Autodesk Inventor part; units mm, degrees
(part 2 of 2)
  line L317 (12.3467, 21.5941) -> (15.1117, 21.5941)
  line L318 (-7.2627, 18.1267) -> (-7.2627, 11.634)
  line L319 (-3.9937, 18.1267) -> (-7.2627, 18.1267)
  line L320 (-3.9937, 11.634) -> (-3.9937, 18.1267)
  line L321 (-7.2627, 11.634) -> (-3.9937, 11.634)
  line L322 (2.8777, 19.9119) -> (2.8777, 17.0508)
  line L323 (5.6982, 19.9119) -> (2.8777, 19.9119)
  line L324 (5.6982, 17.0508) -> (5.6982, 19.9119)
  line L325 (2.8777, 17.0508) -> (5.6982, 17.0508)
  line L326 (6.6317, 14.6767) -> (6.6317, 13.9462)
  line L327 (8.2279, 14.6767) -> (6.6317, 14.6767)
  line L328 (8.2279, 13.9462) -> (8.2279, 14.6767)
  line L329 (6.6317, 13.9462) -> (8.2279, 13.9462)
  line L330 (-11.4396, 26.1143) -> (-11.4396, 21.5941)
  line L331 (-8.2765, 26.1143) -> (-11.4396, 26.1143)
  line L332 (-8.2765, 21.5941) -> (-8.2765, 26.1143)
  line L333 (-11.4396, 21.5941) -> (-8.2765, 21.5941)
  line L334 (23.7979, 4.6422) -> (23.7979, 3.9161)
  line L335 (25.3456, 4.6422) -> (23.7979, 4.6422)
  line L336 (25.3456, 3.9161) -> (25.3456, 4.6422)
  line L337 (23.7979, 3.9161) -> (25.3456, 3.9161)
  line L338 (25.9674, 12.5506) -> (25.9674, 11.0937)
  line L339 (26.969, 12.5506) -> (25.9674, 12.5506)
  line L340 (26.969, 11.0937) -> (26.969, 12.5506)
  line L341 (25.9674, 11.0937) -> (26.969, 11.0937)
  line L342 (20.5866, 13.4064) -> (20.5866, 10.1468)
  line L343 (22.4384, 13.4064) -> (20.5866, 13.4064)
  line L344 (22.4384, 10.1468) -> (22.4384, 13.4064)
  line L345 (20.5866, 10.1468) -> (22.4384, 10.1468)
  line L346 (13.1069, 19.0982) -> (13.1069, 18.337)
  line L347 (14.6707, 19.0982) -> (13.1069, 19.0982)
  line L348 (14.6707, 18.337) -> (14.6707, 19.0982)
  line L349 (13.1069, 18.337) -> (14.6707, 18.337)
  line L350 (-2.8376, 26.8483) -> (-2.8376, 26.1143)
  line L351 (-1.3678, 26.8483) -> (-2.8376, 26.8483)
  line L352 (-1.3678, 26.1143) -> (-1.3678, 26.8483)
  line L353 (-2.8376, 26.1143) -> (-1.3678, 26.1143)
  line L354 (3.5053, 26.9808) -> (3.5053, 26.1143)
  line L355 (5.0811, 26.9808) -> (3.5053, 26.9808)
  line L356 (5.0811, 26.1143) -> (5.0811, 26.9808)
  line L357 (3.5053, 26.1143) -> (5.0811, 26.1143)
  line L358 (9.7366, 26.9808) -> (9.7366, 26.1143)
  line L359 (11.3, 26.9808) -> (9.7366, 26.9808)
  line L360 (11.3, 26.1143) -> (11.3, 26.9808)
  line L361 (9.7366, 26.1143) -> (11.3, 26.1143)
  line L362 (12.7922, 32.175) -> (12.7922, 30.9022)
  line L363 (14.5702, 32.175) -> (12.7922, 32.175)
  line L364 (14.5702, 30.9022) -> (14.5702, 32.175)
  line L365 (12.7922, 30.9022) -> (14.5702, 30.9022)
  line L366 (13.3079, 38.2648) -> (13.3079, 35.0088)
  line L367 (14.1615, 38.2648) -> (13.3079, 38.2648)
  line L368 (14.1615, 35.0088) -> (14.1615, 38.2648)
  line L369 (13.3079, 35.0088) -> (14.1615, 35.0088)
  line L370 (12.9292, 42.1098) -> (12.9292, 41.3551)
  line L371 (14.3655, 42.1098) -> (12.9292, 42.1098)
  line L372 (14.3655, 41.3551) -> (14.3655, 42.1098)
  line L373 (12.9292, 41.3551) -> (14.3655, 41.3551)
  line L374 (-2.9701, 39.8497) -> (-2.9701, 39.0772)
  line L375 (-1.3678, 39.8497) -> (-2.9701, 39.8497)
  line L376 (-1.3678, 39.0772) -> (-1.3678, 39.8497)
  line L377 (-2.9701, 39.0772) -> (-1.3678, 39.0772)
  line L378 (-2.6721, 35.9046) -> (-2.6721, 32.7312)
  line L379 (-1.7091, 35.9046) -> (-2.6721, 35.9046)
  line L380 (-1.7091, 32.7312) -> (-1.7091, 35.9046)
  line L381 (-2.6721, 32.7312) -> (-1.7091, 32.7312)
  line L382 (61.5532, 35.0088) -> (61.5532, 33.5887)
  line L383 (63.3578, 35.0088) -> (61.5532, 35.0088)
  line L384 (63.3578, 33.5887) -> (63.3578, 35.0088)
  line L385 (61.5532, 33.5887) -> (63.3578, 33.5887)
  line L386 (-2.3, 45.1616) -> (-2.3, 41.9097)
  line L387 (-0.4798, 45.1616) -> (-2.3, 45.1616)
  line L388 (-0.4798, 41.9097) -> (-0.4798, 45.1616)
  line L389 (-2.3, 41.9097) -> (-0.4798, 41.9097)
  arc A22 (0.3948, 25.0132) -> (0.3948, 21.2543) centre (0.717, 23.1338) ccw
  line L390 (8.2935, 25.0132) -> (0.3948, 25.0132)
  arc A23 (8.2935, 21.2543) -> (8.2935, 25.0132) centre (7.9713, 23.1338) ccw
  line L391 (0.3948, 21.2543) -> (8.2935, 21.2543)
  circle A24 centre (11.0964, 6.0607) radius 3.302
  line L392 (53.7966, 24.6667) -> (53.7966, 25.3313)
  line L393 (52.7806, 23.6507) -> (53.7966, 24.6667)
  line L394 (49.402, 23.6507) -> (52.7806, 23.6507)
  line L395 (48.386, 24.6667) -> (49.402, 23.6507)
  line L396 (48.386, 25.3313) -> (48.386, 24.6667)
  line L397 (49.402, 26.3473) -> (48.386, 25.3313)
  line L398 (52.7806, 26.3473) -> (49.402, 26.3473)
  line L399 (53.7966, 25.3313) -> (52.7806, 26.3473)
  line L400 (1.7827, 46.235) -> (1.1223, 46.235)
  line L401 (2.7987, 45.219) -> (1.7827, 46.235)
  line L402 (2.7987, 41.8408) -> (2.7987, 45.219)
  line L403 (1.7827, 40.8248) -> (2.7987, 41.8408)
  line L404 (1.1223, 40.8248) -> (1.7827, 40.8248)
  line L405 (0.1063, 41.8408) -> (1.1223, 40.8248)
  line L406 (0.1063, 45.219) -> (0.1063, 41.8408)
  line L407 (1.1223, 46.235) -> (0.1063, 45.219)
  line L408 (6.7103, 46.235) -> (5.6943, 45.219)
  line L409 (7.3707, 46.235) -> (6.7103, 46.235)
  line L410 (8.3867, 45.219) -> (7.3707, 46.235)
  line L411 (8.3867, 41.8408) -> (8.3867, 45.219)
  line L412 (7.3707, 40.8248) -> (8.3867, 41.8408)
  line L413 (6.7103, 40.8248) -> (7.3707, 40.8248)
  line L414 (5.6943, 41.8408) -> (6.7103, 40.8248)
  line L415 (5.6943, 45.219) -> (5.6943, 41.8408)
  circle A25 centre (0, 48.3362) radius 1.5621
  circle A26 centre (0, 0) radius 1.5621
  circle A27 centre (82.6262, 0) radius 1.5621
  circle A28 centre (51.6255, 4.8785) radius 1.5621
  circle A29 centre (51.6255, 32.8947) radius 1.3153
  circle A30 centre (75.1332, 48.3362) radius 1.5621
  line L416 (3.9163, 46.235) -> (2.9003, 45.219)
  line L417 (4.5767, 46.235) -> (3.9163, 46.235)
  line L418 (5.5927, 45.219) -> (4.5767, 46.235)
  line L419 (5.5927, 41.8408) -> (5.5927, 45.219)
  line L420 (4.5767, 40.8248) -> (5.5927, 41.8408)
  line L421 (3.9163, 40.8248) -> (4.5767, 40.8248)
  line L422 (2.9003, 41.8408) -> (3.9163, 40.8248)
  line L423 (2.9003, 45.219) -> (2.9003, 41.8408)
  line L424 (53.7966, 21.8727) -> (53.7966, 22.5373)
  line L425 (52.7806, 20.8567) -> (53.7966, 21.8727)
  line L426 (49.402, 20.8567) -> (52.7806, 20.8567)
  line L427 (48.386, 21.8727) -> (49.402, 20.8567)
  line L428 (48.386, 22.5373) -> (48.386, 21.8727)
  line L429 (49.402, 23.5533) -> (48.386, 22.5373)
  line L430 (52.7806, 23.5533) -> (49.402, 23.5533)
  line L431 (53.7966, 22.5373) -> (52.7806, 23.5533)
  line L432 (53.7966, 27.4607) -> (53.7966, 28.1253)
  line L433 (52.7806, 26.4447) -> (53.7966, 27.4607)
  line L434 (49.402, 26.4447) -> (52.7806, 26.4447)
  line L435 (48.386, 27.4607) -> (49.402, 26.4447)
  line L436 (48.386, 28.1253) -> (48.386, 27.4607)
  line L437 (49.402, 29.1413) -> (48.386, 28.1253)
  line L438 (52.7806, 29.1413) -> (49.402, 29.1413)
  line L439 (53.7966, 28.1253) -> (52.7806, 29.1413)
  circle A31 centre (3.9075, 6.0607) radius 3.302
  line L440 (57.1918, 28.2371) -> (57.1918, 21.9581)
  line L441 (63.6527, 28.2371) -> (57.1918, 28.2371)
  line L442 (63.6527, 21.9581) -> (63.6527, 28.2371)
  line L443 (57.1918, 21.9581) -> (63.6527, 21.9581)
  line L444 (66.3035, 35.9046) -> (66.3035, 32.5006)
  line L445 (67.5508, 35.9046) -> (66.3035, 35.9046)
  line L446 (67.5508, 32.5006) -> (67.5508, 35.9046)
  line L447 (66.3035, 32.5006) -> (67.5508, 32.5006)
  line L448 (-2.9701, 32.0256) -> (-2.9701, 31.0896)
  line L449 (-1.3678, 32.0256) -> (-2.9701, 32.0256)
  line L450 (-1.3678, 31.0896) -> (-1.3678, 32.0256)
  line L451 (-2.9701, 31.0896) -> (-1.3678, 31.0896)
  line L452 (-2.9701, 37.5322) -> (-2.9701, 36.6368)
  line L453 (-1.3678, 37.5322) -> (-2.9701, 37.5322)
  line L454 (-1.3678, 36.6368) -> (-1.3678, 37.5322)
  line L455 (-2.9701, 36.6368) -> (-1.3678, 36.6368)
  line L456 (-6.9964, 42.9992) -> (-6.9964, 41.9097)
  line L457 (-5.0545, 42.9992) -> (-6.9964, 42.9992)
  line L458 (-5.0545, 41.9097) -> (-5.0545, 42.9992)
  line L459 (-6.9964, 41.9097) -> (-5.0545, 41.9097)
  line L460 (12.7922, 40.0541) -> (12.7922, 38.8221)
  line L461 (14.5702, 40.0541) -> (12.7922, 40.0541)
  line L462 (14.5702, 38.8221) -> (14.5702, 40.0541)
  line L463 (12.7922, 38.8221) -> (14.5702, 38.8221)
  line L464 (12.7922, 34.4881) -> (12.7922, 33.2287)
  line L465 (14.5702, 34.4881) -> (12.7922, 34.4881)
  line L466 (14.5702, 33.2287) -> (14.5702, 34.4881)
  line L467 (12.7922, 33.2287) -> (14.5702, 33.2287)
  line L468 (13.3079, 29.9286) -> (13.3079, 26.7098)
  line L469 (14.3655, 29.9286) -> (13.3079, 29.9286)
  line L470 (14.3655, 26.7098) -> (14.3655, 29.9286)
  line L471 (13.3079, 26.7098) -> (14.3655, 26.7098)
  line L472 (6.6317, 26.9808) -> (6.6317, 26.1143)
  line L473 (8.1119, 26.9808) -> (6.6317, 26.9808)
  line L474 (8.1119, 26.1143) -> (8.1119, 26.9808)
  line L475 (6.6317, 26.1143) -> (8.1119, 26.1143)
  line L476 (0.2905, 26.8483) -> (0.2905, 26.1143)
  line L477 (1.8236, 26.8483) -> (0.2905, 26.8483)
  line L478 (1.8236, 26.1143) -> (1.8236, 26.8483)
  line L479 (0.2905, 26.1143) -> (1.8236, 26.1143)
  line L480 (-2.9701, 28.4771) -> (-2.9701, 27.8018)
  line L481 (-1.3678, 28.4771) -> (-2.9701, 28.4771)
  line L482 (-1.3678, 27.8018) -> (-1.3678, 28.4771)
  line L483 (-2.9701, 27.8018) -> (-1.3678, 27.8018)
  line L484 (13.0148, 15.7926) -> (13.0148, 15.0444)
  line L485 (14.5702, 15.7926) -> (13.0148, 15.7926)
  line L486 (14.5702, 15.0444) -> (14.5702, 15.7926)
  line L487 (13.0148, 15.0444) -> (14.5702, 15.0444)
  line L488 (23.6729, 13.4064) -> (23.6729, 10.1468)
  line L489 (24.9476, 13.4064) -> (23.6729, 13.4064)
  line L490 (24.9476, 10.1468) -> (24.9476, 13.4064)
  line L491 (23.6729, 10.1468) -> (24.9476, 10.1468)
  line L492 (18.9382, 13.024) -> (18.9382, 10.8934)
  line L493 (19.9033, 13.024) -> (18.9382, 13.024)
  line L494 (19.9033, 10.8934) -> (19.9033, 13.024)
  line L495 (18.9382, 10.8934) -> (19.9033, 10.8934)
  line L496 (-5.6282, 24.3602) -> (-5.6282, 21.5941)
  line L497 (-4.4808, 24.3602) -> (-5.6282, 24.3602)
  line L498 (-4.4808, 21.5941) -> (-4.4808, 24.3602)
  line L499 (-5.6282, 21.5941) -> (-4.4808, 21.5941)
  line L500 (-0.1051, 15.5086) -> (-0.1051, 13.9462)
  line L501 (0.6862, 15.5086) -> (-0.1051, 15.5086)
  line L502 (0.6862, 13.9462) -> (0.6862, 15.5086)
  line L503 (-0.1051, 13.9462) -> (0.6862, 13.9462)
  line L504 (3.872, 15.2448) -> (3.872, 12.0387)
  line L505 (4.8257, 15.2448) -> (3.872, 15.2448)
  line L506 (4.8257, 12.0387) -> (4.8257, 15.2448)
  line L507 (3.872, 12.0387) -> (4.8257, 12.0387)
  line L508 (5.5046, 1.1225) -> (5.5046, -1.3243)
  line L509 (9.5396, 1.1225) -> (5.5046, 1.1225)
  line L510 (9.5396, -1.3243) -> (9.5396, 1.1225)
  line L511 (5.5046, -1.3243) -> (9.5396, -1.3243)
  line L512 (3.1684, 34.4881) -> (3.1684, 29.563)
  line L513 (8.2279, 34.4881) -> (3.1684, 34.4881)
  line L514 (8.2279, 29.563) -> (8.2279, 34.4881)
  line L515 (3.1684, 29.563) -> (8.2279, 29.563)
  line L516 (29.7171, 32.7312) -> (29.7171, 18.5332)
  line L517 (43.7506, 32.7312) -> (29.7171, 32.7312)
  line L518 (43.7506, 18.5332) -> (43.7506, 32.7312)
  line L519 (29.7171, 18.5332) -> (43.7506, 18.5332)
  circle A32 centre (0, 0) radius 1.25
  circle A33 centre (0, 48.3362) radius 1.25
  circle A34 centre (51.6255, 4.8785) radius 2.5
  circle A35 centre (51.6255, 4.8785) radius 1.1
  circle A36 centre (51.6255, 32.8947) radius 1
  circle A37 centre (75.1332, 48.3362) radius 1.25
  circle A38 centre (82.6262, 0) radius 1.25
  point P0 (-14.1224, -2.54)
  dimension "d11" = 2.5
  dimension "d12" = 2.5
  dimension "d13" = 2.2
  dimension "d14" = 2
  dimension "d15" = 2.5
  dimension "d16" = 2.5
  constraints: 6 centre point, 6 coincident
  measures "d11" diameter of A32
  measures "d12" diameter of A33
  measures "d13" diameter of A35
  measures "d14" diameter of A36
  measures "d15" diameter of A37
  measures "d16" diameter of A38
extrude "Vysunutí3" add sketch "Náčrt3" along normal blind 2 contours A35 | A36 | A37 | A38
sketch "Náčrt4" plane through (0, 0, 2) normal (0, 0, 1) x (1, 0, 0)
  line L0 (-101.6, 53.4162) -> (-101.6, 0)
  line L1 (-101.6, 0) -> (0, 0)
  line L2 (0, 0) -> (0, 53.4162)
  line L3 (0, 53.4162) -> (-101.6, 53.4162)
  line L4 (0, 66.8994) -> (0, -13.4832)
  line L5 (-124.72, 0) -> (23.12, 0)
  line L6 (-103.6, 55.4162) -> (-103.6, -2)
  line L7 (-103.6, -2) -> (2, -2)
  line L8 (2, -2) -> (2, 55.4162)
  line L9 (2, 55.4162) -> (-103.6, 55.4162)
  dimension "d19" = 2
  constraints: 8 end point, 3 other
  measures "d19" distance between parallel lines of L3 L9
extrude "Vysunutí4" add sketch "Náčrt4" against normal up to surface (2 mm away)
sketch "Náčrt5" plane through (0, 0, 2) normal (0, 0, 1) x (1, 0, 0)
  line L0 (2, -2) -> (2, 55.4162)
  line L1 (2, 55.4162) -> (-103.6, 55.4162)
  line L2 (-103.6, 55.4162) -> (-103.6, -2)
  line L3 (-103.6, -2) -> (2, -2)
  line L4 (0, 71.0994) -> (0, -17.6832)
  line L5 (-128.92, 0) -> (27.32, 0)
  line L6 (5, -5) -> (-106.6, -5)
  line L7 (-106.6, -5) -> (-106.6, 58.4162)
  line L8 (-106.6, 58.4162) -> (5, 58.4162)
  line L9 (-103.6, -2) -> (2, -2)
  line L10 (2, -2) -> (2, 55.4162)
  line L11 (2, 55.4162) -> (-103.6, 55.4162)
  line L12 (-103.6, 55.4162) -> (-103.6, -2)
  line L13 (5, -5) -> (5, 58.4162)
  line L14 (-103.6, 55.4162) -> (2, 55.4162)
  line L15 (2, 55.4162) -> (2, -2)
  line L16 (2, -2) -> (-103.6, -2)
  line L17 (-103.6, -2) -> (-103.6, 55.4162)
  circle A0 centre (-89.2556, 50.8762) radius 2.5
  circle A1 centre (-14.1224, 2.54) radius 2.5
  circle A2 centre (-96.7486, 2.54) radius 2.5
  circle A3 centre (-65.7479, 35.4347) radius 2.5
  circle A4 centre (-14.1224, 50.8762) radius 2.5
  circle A5 centre (-65.7479, 7.4185) radius 2.5
  point P0 (0, 0)
  dimension "d29" = 3
  dimension "d30" = 3
  constraints: 16 end point, 2 parallel, 1 horizontal, 1 perpendicular, 1 vertical, 2 other
  measures "d29" distance between parallel lines of L0 L13
  measures "d30" distance between parallel lines of L1 L8
extrude "Vysunutí5" add sketch "Náčrt5" against normal blind 15 contours L0 L5 L13 L6 L4 L3 | L0 L1 L4 L8 L13 L5 | L4 L6 L7 L5 L2 L3 | L1 L2 L5 L7 L8 L4
fillet "Zaoblení1" radius 2 4 edges at (5, 58.4162, -5.5) (5, -5, -5.5) (-106.6, -5, -5.5) (-106.6, 58.4162, -5.5)
sketch "Náčrt7" plane through (5, -3, 2) normal (1, 0, 0) x (0, 0, -1)
  line L0 (15, 58.4162) -> (15, 1)
  line L1 (15, 48.6662) -> (6.551, 48.6662)
  line L2 (6.551, 48.6662) -> (6.551, 35.6662)
  line L3 (6.551, 35.6662) -> (15, 35.6662)
  line L4 (15, 35.6662) -> (15, 48.6662)
  line L5 (15, 0) -> (0, 0)
  line L6 (15, 59.4162) -> (15, 0)
  line L7 (0, 59.4162) -> (15, 59.4162)
  line L8 (0, 0) -> (0, 59.4162)
  line L9 (15, 61.4162) -> (0, 61.4162)
  line L10 (15, 19.75) -> (6.501, 19.75)
  line L11 (6.501, 19.75) -> (6.501, 9.75)
  line L12 (6.501, 9.75) -> (15, 9.75)
  line L13 (15, 9.75) -> (15, 19.75)
  line L14 (0, -2) -> (15, -2)
  point P0 (2, 3)
  point P1 (15, 9.75)
  point P2 (15, 35.6662)
  dimension "d32" = 13
  dimension "d33" = 6.551
  dimension "d37" = 8.499
  dimension "d40" = 10
  dimension "d45" = 10.75
  dimension "d46" = 9.75
  constraints: 16 end point, 4 parallel, 2 horizontal, 2 perpendicular, 2 point on line
  measures "d32" distance of L1.end L2.end
  measures "d33" distance between parallel lines of L8 L2
  measures "d37" distance between parallel lines of L0 L11
  measures "d40" distance between parallel lines of L12 L10
  measures "d45" distance between parallel lines of L7 L1
  measures "d46" distance between parallel lines of L5 L12
extrude "Vysunutí7" cut sketch "Náčrt7" against normal up to surface (3 mm away) contours L0 L3 L2 L1 | L0 L12 L11 L10
ref_plane "Pracovní rovina1" through (0, 0, -7) normal (0, 0, -1) x (-1, 0, 0)
sketch "Náčrt8" plane through (0, 0, -13) normal (0, 0, -1) x (-1, 0, 0)
  line L0 (-2, 6.75) -> (-5, 6.75)
  line L1 (-5, 6.75) -> (-5, -3)
  arc A0 (-5, -3) -> (-3, -5) centre (-3, -3) ccw
  line L2 (-3, -5) -> (104.6, -5)
  arc A1 (104.6, -5) -> (106.6, -3) centre (104.6, -3) ccw
  line L3 (106.6, -3) -> (106.6, 56.4162)
  arc A2 (106.6, 56.4162) -> (104.6, 58.4162) centre (104.6, 56.4162) ccw
  line L4 (104.6, 58.4162) -> (-3, 58.4162)
  arc A3 (-3, 58.4162) -> (-5, 56.4162) centre (-3, 56.4162) ccw
  line L5 (-5, 56.4162) -> (-5, 45.6662)
  line L6 (-5, 45.6662) -> (-2, 45.6662)
  line L7 (-2, 45.6662) -> (-2, 55.4162)
  line L8 (-2, 55.4162) -> (103.6, 55.4162)
  line L9 (103.6, 55.4162) -> (103.6, -2)
  line L10 (103.6, -2) -> (-2, -2)
  line L11 (-2, -2) -> (-2, 6.75)
  line L12 (-3, 58.4162) -> (104.6, 58.4162)
  arc A4 (106.6, 56.4162) -> (104.6, 58.4162) centre (104.6, 56.4162) ccw
  line L13 (106.6, 56.4162) -> (106.6, -3)
  arc A5 (104.6, -5) -> (106.6, -3) centre (104.6, -3) ccw
  line L14 (104.6, -5) -> (-3, -5)
  arc A6 (-5, -3) -> (-3, -5) centre (-3, -3) ccw
  line L15 (-5, -3) -> (-5, 6.75)
  line L16 (-5, 6.75) -> (-2, 6.75)
  line L17 (-2, 6.75) -> (-2, -2)
  line L18 (-2, -2) -> (103.6, -2)
  line L19 (103.6, -2) -> (103.6, 55.4162)
  line L20 (103.6, 55.4162) -> (-2, 55.4162)
  line L21 (-2, 55.4162) -> (-2, 45.6662)
  line L22 (-2, 45.6662) -> (-5, 45.6662)
  line L23 (-5, 45.6662) -> (-5, 56.4162)
  arc A7 (-3, 58.4162) -> (-5, 56.4162) centre (-3, 56.4162) ccw
  line L24 (-5, 16.75) -> (-2, 16.75)
  line L25 (-2, 16.75) -> (-2, 32.6662)
  line L26 (-2, 32.6662) -> (-5, 32.6662)
  line L27 (-5, 32.6662) -> (-5, 16.75)
  line L28 (-2, 32.6662) -> (-2, 16.75)
  line L29 (-2, 16.75) -> (-5, 16.75)
  line L30 (-5, 16.75) -> (-5, 32.6662)
  line L31 (-5, 32.6662) -> (-2, 32.6662)
  point P0 (0, 0)
  dimension "d48" = 0
  dimension "d49" = 0
  constraints: 32 end point, 8 point on circle, 4 centre point, 18 other
  measures "d48" distance between parallel lines of L26 L31
  measures "d49" distance between parallel lines of L6 L22
extrude "Vysunutí8" add sketch "Náčrt8" along normal blind 5
sketch "Náčrt9" plane through (0, 0, 2) normal (0, 0, 1) x (1, 0, 0)
  arc A0 (-104.6, 58.4162) -> (-106.6, 56.4162) centre (-104.6, 56.4162) ccw
  line L0 (-106.6, 56.4162) -> (-106.6, -3)
  arc A1 (-106.6, -3) -> (-104.6, -5) centre (-104.6, -3) ccw
  line L1 (-104.6, -5) -> (3, -5)
  arc A2 (3, -5) -> (5, -3) centre (3, -3) ccw
  line L2 (5, -3) -> (5, 56.4162)
  arc A3 (5, 56.4162) -> (3, 58.4162) centre (3, 56.4162) ccw
  line L3 (3, 58.4162) -> (-104.6, 58.4162)
  line L4 (5, 21.708) -> (15, 21.708)
  line L5 (15, 21.708) -> (15, 31.708)
  line L6 (15, 31.708) -> (5, 31.708)
  line L7 (5, 31.708) -> (5, 21.708)
  point P0 (0, 0)
  point P1 (5, 31.708)
  dimension "d52" = 10
  dimension "d53" = 10
  dimension "d54" = 26.708
  constraints: 8 end point, 2 parallel, 1 horizontal, 1 perpendicular, 1 point on line
  measures "d52" distance of L6.end L5.end
  measures "d53" distance of L5.end L4.end
  measures "d54" distance between parallel lines of L1 L4
extrude "Vysunutí9" add sketch "Náčrt9" against normal blind 4 contours L6 L5 L4 L2
sketch "Náčrt10" plane through (0, 0, -2) normal (0, 0, -1) x (-1, 0, 0)
  line L0 (-5, 31.708) -> (-15, 31.708)
  line L1 (-15, 31.708) -> (-15, 21.708)
  line L2 (-15, 21.708) -> (-5, 21.708)
  line L3 (-5, 31.708) -> (-5, 21.708)
  point P0 (0, 0)
  point P1 (-10, 26.708)
  dimension "d57" = 5
  dimension "d58" = 5
  measures "d57" distance from line of L0 point (-10, 26.708)
  measures "d58" distance from line of L1 point (-10, 26.708)
hole "Díra1" at (10, 26.708, -2) direction (0, 0, 1) diameter 5 end through all
fillet "Zaoblení2" radius 2 2 edges at (15, 31.708, 0) (15, 21.708, 0)
ref_plane "Pracovní rovina2" through (-50.8, 32.6662, -4.551) normal (1, 0, 0) x (0, 0, -1)
mirror "Zrcadlit1" about plane through (-50.8, 32.6662, -4.551) normal (1, 0, 0) of "Díra1", "Vysunutí9", "Zaoblení2"
